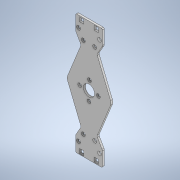
# Autodesk Inventor part: Ось
Saved by Autodesk Inventor 2021 (Build 250183000, 183)
## iProperties
Created: 2022-07-08
Part Number: Ось
Material: Типовые
Document SubType Name: Modeling
Designer: zvi20
Density: 1 g/cm^3
Appearance: По умолчанию
Author: zvi20
Autodesk Inventor part; units mm, degrees
ref_plane "YZ Plane" through (0, 0, 0) normal (1, 0, 0) x (0, 1, 0)
ref_plane "XZ Plane" through (0, 0, 0) normal (0, 1, 0) x (-1, 0, 0)
ref_plane "XY Plane" through (0, 0, 0) normal (0, 0, 1) x (1, 0, 0)
sketch "Эскиз1" plane through (0, 0, 0) normal (0, 0, 1) x (1, 0, 0)
  arc A0 (18.8037, 34.9783) -> (30.573, 34.9783) centre (24.6884, 34.9783) ccw
  arc A1 (12.9191, 34.9783) -> (16.8422, 34.9783) centre (14.8807, 34.9783) ccw
  circle A2 centre (24.6884, 25.1706) radius 1.9615
  arc A3 (32.5345, 34.9783) -> (36.4576, 34.9783) centre (34.4961, 34.9783) ccw
  line L0 (47.3356, 32.8988) -> (33.4131, -1.4608)
  line L1 (15.9516, -1.4608) -> (2.0291, 32.8988)
  arc A4 (30.573, 34.9783) -> (18.8037, 34.9783) centre (24.6884, 34.9783) ccw
  arc A5 (16.8422, 34.9783) -> (12.9191, 34.9783) centre (14.8807, 34.9783) ccw
  circle A6 centre (25.1823, 44.7322) radius 1.9615
  arc A7 (36.4576, 34.9783) -> (32.5345, 34.9783) centre (34.4961, 34.9783) ccw
  arc A8 (47.3356, 32.8988) -> (47.3356, 37.0577) centre (42.2036, 34.9783) ccw
  arc A9 (2.0291, 37.0577) -> (2.0291, 32.8988) centre (7.161, 34.9783) ccw
  line L2 (24.6823, -28.3537) -> (11.6823, -28.3537)
  line L3 (10.6823, -27.3537) -> (10.6823, -13.1403)
  line L4 (11.0683, -11.6683) -> (15.8407, -3.1932)
  arc A10 (11.0683, -11.6683) -> (10.6823, -13.1403) centre (13.6823, -13.1403) ccw
  arc A11 (10.6823, -27.3537) -> (11.6823, -28.3537) centre (11.6823, -27.3537) ccw
  line L5 (38.6823, -26.8537) -> (38.6823, -13.1403)
  line L6 (38.2964, -11.6683) -> (33.524, -3.1932)
  arc A12 (38.6823, -13.1403) -> (38.2964, -11.6683) centre (35.6823, -13.1403) ccw
  arc A13 (15.8407, -3.1932) -> (15.9516, -1.4608) centre (14.098, -2.2119) ccw
  arc A14 (33.4131, -1.4608) -> (33.524, -3.1932) centre (35.2667, -2.2119) ccw
  line L7 (14.6823, -27.3537) -> (19.1823, -27.3537)
  line L8 (19.1823, -27.3537) -> (19.1823, -22.8537)
  line L9 (19.1823, -22.8537) -> (14.6823, -22.8537)
  line L10 (14.6823, -22.8537) -> (14.6823, -27.3537)
  circle A15 centre (13.6823, -16.8537) radius 2
  circle A16 centre (18.6823, -7.8537) radius 2
  line L11 (38.6823, -26.8537) -> (38.6823, -27.3537)
  line L12 (24.6823, -28.3537) -> (37.6823, -28.3537)
  arc A17 (37.6823, -28.3537) -> (38.6823, -27.3537) centre (37.6823, -27.3537) ccw
  line L13 (34.6823, -27.3537) -> (30.1823, -27.3537)
  line L14 (30.1823, -27.3537) -> (30.1823, -22.8537)
  line L15 (30.1823, -22.8537) -> (34.6823, -22.8537)
  line L16 (34.6823, -22.8537) -> (34.6823, -27.3537)
  circle A18 centre (35.6823, -16.8537) radius 2
  circle A19 centre (30.6823, -7.8537) radius 2
  line L17 (47.3356, 37.0577) -> (33.4131, 71.4174)
  line L18 (15.9516, 71.4174) -> (2.0291, 37.0577)
  line L19 (24.6823, 98.3103) -> (11.6823, 98.3103)
  line L20 (10.6823, 97.3103) -> (10.6823, 83.0969)
  line L21 (11.0683, 81.6249) -> (15.8407, 73.1498)
  arc A20 (10.6823, 83.0969) -> (11.0683, 81.6249) centre (13.6823, 83.0969) ccw
  arc A21 (11.6823, 98.3103) -> (10.6823, 97.3103) centre (11.6823, 97.3103) ccw
  line L22 (38.2964, 81.6249) -> (33.524, 73.1498)
  arc A22 (38.2964, 81.6249) -> (38.6823, 83.0969) centre (35.6823, 83.0969) ccw
  line L23 (38.6823, 96.8103) -> (38.6823, 83.0969)
  arc A23 (15.9516, 71.4174) -> (15.8407, 73.1498) centre (14.098, 72.1684) ccw
  arc A24 (33.524, 73.1498) -> (33.4131, 71.4174) centre (35.2667, 72.1684) ccw
  line L24 (14.6823, 97.3103) -> (19.1823, 97.3103)
  line L25 (19.1823, 97.3103) -> (19.1823, 92.8103)
  line L26 (19.1823, 92.8103) -> (14.6823, 92.8103)
  line L27 (14.6823, 92.8103) -> (14.6823, 97.3103)
  circle A25 centre (13.6823, 86.8103) radius 2
  circle A26 centre (18.6823, 77.8103) radius 2
  line L28 (38.6823, 96.8103) -> (38.6823, 97.3103)
  line L29 (24.6823, 98.3103) -> (37.6823, 98.3103)
  arc A27 (38.6823, 97.3103) -> (37.6823, 98.3103) centre (37.6823, 97.3103) ccw
  circle A28 centre (30.6823, 77.8103) radius 2
  circle A29 centre (35.6823, 86.8103) radius 2
  line L30 (30.1823, 92.8103) -> (34.6823, 92.8103)
  line L31 (30.1823, 97.3103) -> (30.1823, 92.8103)
  line L32 (34.6823, 97.3103) -> (30.1823, 97.3103)
  line L33 (34.6823, 92.8103) -> (34.6823, 97.3103)
  point P0 (0, 0)
  point P1 (10.6823, -12.3537)
  point P2 (38.6823, -12.3537)
  point P3 (10.6823, 82.3103)
  point P4 (38.6823, 82.3103)
  dimension "d89" = 9
  dimension "d91" = 5
  dimension "d93" = 3
  dimension "d94" = 4
  dimension "d95" = 4
  dimension "d98" = 4.5
  dimension "d99" = 4.5
  dimension "d100" = 6
  dimension "d105" = 1
  constraints: 68 end point, 40 point on circle, 30 centre point, 12 tangent, 8 point on line, 3 horizontal, 2 parallel, 2 vertical, 1 perpendicular
  measures "d89" vertical distance of A16.centre A15.centre
  measures "d91" horizontal distance of A15.centre A16.centre
  measures "d93" distance from line of A15.centre L3
  measures "d94" diameter of A15
  measures "d95" diameter of A16
  measures "d98" distance of L7.end L8.end
  measures "d99" distance of L8.end L9.end
  measures "d100" distance from line of L9 A15.centre
  measures "d105" distance between parallel lines of L2 L7
extrude "Выдавливание3" add sketch "Эскиз1" along normal blind 2
